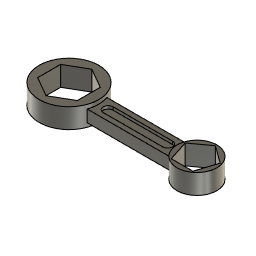
Practice2 (Autodesk Fusion 360 design; units mm, degrees)
Autodesk Fusion 360 part; units mm, degrees
sketch "Sketch1" plane through (0, 0, 0) normal (0, 0, 1) x (1, 0, 0)
  circle A0 centre (0, 0) radius 30
  circle A1 centre (129, 0) radius 20
  line L0 (0, 23.094) -> (-20, 11.547)
  line L1 (-20, 11.547) -> (-20, -11.547)
  line L2 (-20, -11.547) -> (0, -23.094)
  line L3 (0, -23.094) -> (20, -11.547)
  line L4 (20, -11.547) -> (20, 11.547)
  line L5 (20, 11.547) -> (0, 23.094)
  line L6 (146.6336, 5.7295) -> (129, 18.541)
  line L7 (129, 18.541) -> (111.3664, 5.7295)
  line L8 (111.3664, 5.7295) -> (118.1019, -15)
  line L9 (118.1019, -15) -> (139.8981, -15)
  line L10 (139.8981, -15) -> (146.6336, 5.7295)
  line L11 (28.2843, 10) -> (111.6795, 10)
  line L12 (28.2843, -10) -> (111.6795, -10)
  line L13 (99.5, 5) -> (39.5, 5)
  line L14 (39.5, -5) -> (99.5, -5)
  arc A2 (39.5, 5) -> (39.5, -5) centre (39.5, 0) ccw
  arc A3 (99.5, -5) -> (99.5, 5) centre (99.5, 0) ccw
  point P0 (129, 0)
  point P1 (69.5, 0)
  dimension "d2" = 129
  dimension "d4" = 20
  dimension "d5" = 60
  dimension "d6" = 15
  dimension "d7" = 40
  dimension "d8" = 60
  dimension "d9" = 10
  dimension "d11" = 10
  dimension "d12" = 20
  constraint coincident A0.centre origin
  constraint vertical L1
  constraint coincident P0 A1.centre
  constraint horizontal L9
  constraint horizontal L11
  constraint horizontal L12
  constraint coincident A0 L11.start
  constraint coincident A0 L12.start
  constraint coincident A1 L11.end
  constraint coincident A1 L12.end
  constraint horizontal L13
  constraint parallel L13 L14
  constraint tangent L14 A2
  measures "d2" distance of A0.centre A1.centre
  measures "d4" distance of A0.centre L5
  measures "d5" diameter of A0
  measures "d6" distance of P0 L10
  measures "d7" diameter of A1
  measures "d8" distance of L14.start L14.end
  measures "d9" distance of L13.end L14.start
  measures "d11" distance of L13 L14
  measures "d12" distance of L11 L12
extrude "Extrude1" add sketch "Sketch1" along normal mid plane 20 contours A0 | A1 makes body 1 at (148.9006, -1.9914, -3.3333) makes body 2 at (27.1662, -12.7278, 3.3333)
extrude "Extrude2" add sketch "Sketch1" along normal mid plane 12 contours A0 A1 L11 L12 bodies 1 2
extrude "Extrude3" add sketch "Sketch1" along normal mid plane 6 contours L13 L14 A2 A3 bodies 1
